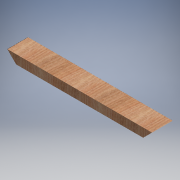
# Autodesk Inventor part: Short Wall 45 Diagonal Piece
Saved by Autodesk Inventor 2016 (Build 200138000, 138)
## iProperties
Created: 2015-07-05
Part Number: Short Wall 45 Diagonal Piece
Material: Wood (Birch)
Document SubType Name: Modeling
Designer: steele
Density: 0.55 g/cm^3
Appearance: Birch - Natural Polished
Author: steele
Autodesk Inventor part; units mm, degrees
ref_plane "YZ Plane" through (0, 0, 0) normal (1, 0, 0) x (0, 1, 0)
ref_plane "XZ Plane" through (0, 0, 0) normal (0, 1, 0) x (-1, 0, 0)
ref_plane "XY Plane" through (0, 0, 0) normal (0, 0, 1) x (1, 0, 0)
sketch "Sketch2" plane through (0, 0, 0) normal (0, 0, 1) x (1, 0, 0)
  line L0 (-288.7165, -19.9295) -> (270.0835, -19.9295)
  line L1 (308.1835, 18.1705) -> (-326.8165, 18.1705)
  line L2 (-272.6622, -16.0762) -> (308.1835, 18.1705) construction
  line L3 (254.1408, -14.1298) -> (-326.8165, 18.1705) construction
  line L4 (-326.8165, 18.1705) -> (-288.7165, -19.9295)
  line L5 (-326.8165, 18.1705) -> (-272.9349, 18.1705) construction
  line L6 (308.1835, 18.1705) -> (270.0835, -19.9295)
  line L7 (308.1835, 18.1705) -> (362.0651, 18.1705) construction
  point P0 (0, 0)
  dimension "d10" = 45
  dimension "d11" = 135
  dimension "d14" = 635
  dimension "d15" = 38.1
  constraints: 16 end point, 3 horizontal, 2 equal length, 2 point on line, 1 parallel
  measures "d10" angle of L4 L5
  measures "d11" angle of L6 L7
  measures "d14" distance of L1.start L1.end
  measures "d15" distance between parallel lines of L0 L1
extrude "Extrusion2" add sketch "Sketch2" along normal mid plane 88.9
body "Solid2"
